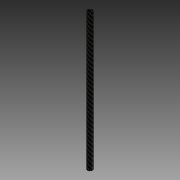
# Autodesk Inventor part: ROD003 - Rod 9.5mm
Saved by Autodesk Inventor 2015 SP1 (Build 190203100, 203)
## iProperties
Created: 2015-05-12
Part Number: ROD003 - Rod 9.5mm
Material: Generic
Document SubType Name: Modeling
Designer: rhornbak
Density: 1 g/cm^3
Appearance: Default
Author: rhornbak
Autodesk Inventor part; units mm, degrees
ref_plane "YZ Plane" through (0, 0, 0) normal (1, 0, 0) x (0, 1, 0)
ref_plane "XZ Plane" through (0, 0, 0) normal (0, 1, 0) x (-1, 0, 0)
ref_plane "XY Plane" through (0, 0, 0) normal (0, 0, 1) x (1, 0, 0)
sketch "Sketch1" plane through (0, 0, 0) normal (0, 0, 1) x (1, 0, 0)
  circle A0 centre (0, 0) radius 4.225
  circle A1 centre (0, 0) radius 4.775
  dimension "RodInner" = 8.45
  dimension "RodDia" = 9.55
  constraints: 2 centre point, 2 coincident
  measures "RodInner" diameter of A0
  measures "RodDia" diameter of A1
extrude "Extrusion1" add sketch "Sketch1" along normal mid plane 250
body "Solid1"
